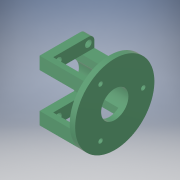
# Autodesk Inventor part: AS5047DEnclosure
Saved by Autodesk Inventor 2019.1 (Build 231200000, 200)
## iProperties
Created: 2018-06-30
Part Number: AS5047DEnclosure
Material: Generisch
Document SubType Name: Modeling
Designer: JochenAlt
Density: 1 g/cm^3
Appearance: Glatt - dunkelseegrün
Author: JochenAlt
Autodesk Inventor part; units mm, degrees
ref_plane "YZ Plane" through (0, 0, 0) normal (1, 0, 0) x (0, 1, 0)
ref_plane "XZ Plane" through (0, 0, 0) normal (0, 1, 0) x (-1, 0, 0)
ref_plane "XY Plane" through (0, 0, 0) normal (0, 0, 1) x (1, 0, 0)
ref_plane "Arbeitsebene1" through (0, 0, 0) normal (1, 0, 0) x (0, 0, -1)
sketch "Skizze1" plane through (0, 0, 0) normal (1, 0, 0) x (0, 0, -1)
  arc A0 (14.55, 0) -> (-14.55, 0) centre (0, 0) ccw
  circle A1 centre (0, 0) radius 5
  line L0 (-20.8128, 0) -> (22.3238, 0) construction
  line L1 (0, -22.3037) -> (0, 20.6923) construction
  circle A2 centre (0, 10.45) radius 0.8
  circle A3 centre (-9.05, -5.225) radius 0.8
  circle A4 centre (9.05, -5.225) radius 0.8
  circle A5 centre (0, 0) radius 10.45 construction
  line L2 (0, 0) -> (9.05, -5.225) construction
  line L3 (0, 0) -> (-9.05, -5.225) construction
  line L4 (8.89, -5.5) -> (-8.89, -5.5) construction
  line L5 (-8.89, -5.5) -> (-8.89, 5.5) construction
  line L6 (-8.89, 5.5) -> (8.89, 5.5) construction
  line L7 (8.89, 5.5) -> (8.89, -5.5) construction
  circle A6 centre (8.89, 5.5) radius 1.2
  circle A7 centre (-8.89, 5.5) radius 1.2
  arc A8 (-14.55, 0) -> (14.1469, 3.4013) centre (0, 0) ccw
  line L8 (8.89, 7.7) -> (-8.89, 7.7)
  line L9 (6.5, 3.3) -> (6.5, 7.7)
  line L10 (-4.3414, 8.5633) -> (-4.3414, 8.4781)
  line L11 (-6.5, 7.7) -> (-6.5, 3.3)
  arc A9 (3.7563, 3.3) -> (-3.7563, 3.3) centre (0, 0) ccw
  line L12 (6.5, 3.3) -> (3.7563, 3.3)
  line L13 (-3.7563, 3.3) -> (-6.5, 3.3)
  line L14 (-6.5, -9.4188) -> (-6.5, -7.4188)
  line L15 (6.5, -9.4188) -> (6.5, -7.4188)
  line L16 (11.09, -9.4188) -> (6.5, -9.4188)
  line L17 (11.09, -9.4188) -> (11.09, -7.4188)
  circle A10 centre (8.89, -5.5) radius 1.2
  circle A11 centre (-8.89, -5.5) radius 1.2
  line L18 (11.09, -7.4188) -> (11.09, 5.5)
  line L19 (-6.5, -7.4188) -> (-6.5, 3.3)
  line L20 (-11.09, -7.4188) -> (-11.09, 5.5)
  arc A12 (-8.89, 7.7) -> (-11.09, 5.5) centre (-8.89, 5.5) ccw
  arc A13 (11.09, 5.5) -> (8.89, 7.7) centre (8.89, 5.5) ccw
  arc A14 (7.715, -7.4188) -> (10.065, -7.4188) centre (8.89, -5.5) ccw
  line L21 (6.5, -7.4188) -> (7.715, -7.4188)
  line L22 (10.065, -7.4188) -> (11.09, -7.4188)
  arc A15 (-10.065, -7.4188) -> (-7.715, -7.4188) centre (-8.89, -5.5) ccw
  line L23 (-11.09, -7.4188) -> (-10.065, -7.4188)
  line L24 (-7.715, -7.4188) -> (-6.5, -7.4188)
  line L25 (6.5, -7.4188) -> (6.5, 3.3)
  line L26 (-11.09, -7.4188) -> (-11.09, -9.4188)
  line L27 (-11.09, -9.4188) -> (-6.5, -9.4188)
  point P0 (0, 14.55)
  dimension "d2" = 10
  dimension "d9" = 1.6
  dimension "d11" = 120
  dimension "d12" = 20.9
  dimension "d19" = 11
  dimension "d20" = 17.78
  dimension "d22" = 2.4
  dimension "d29" = 14.55
  dimension "d30" = 5
  dimension "d38" = 2.2
  dimension "d39" = 13
  dimension "d41" = 2
  dimension "d42" = 4.5
  constraints: 53 end point, 23 point on circle, 16 centre point, 13 coincident, 8 perpendicular, 8 point on line, 7 collinear, 7 equal radius, 6 parallel, 4 tangent, 3 horizontal, 3 vertical, 1 symmetric about line, 6 other
  measures "d2" diameter of A1
  measures "d9" diameter of A2
  measures "d11" angle of L2 L1
  measures "d12" diameter of A5
  measures "d19" distance of L4.end L5.end
  measures "d20" distance of L5.end L6.end
  measures "d22" diameter of A6
  measures "d29" radius of A8
  measures "d30" radius of A9
  measures "d38" radius of A12
  measures "d39" distance between parallel lines of L9 L11
  measures "d41" distance between parallel lines of L22 L16
  measures "d42" diameter of A14
extrude "Extrusion1" add sketch "Skizze1" against normal blind 2 contours A8 L17 L18 A13 L8 A12 L20 L26 A0 | A8 L27 L14 L19 L13 A1 L12 L25 L15 L16 | L16 L15 L21 A14 L22 L17 | L26 L23 A15 L24 L14 L27 | L22 A14 L21 L25 L9 L8 A13 L18 | L20 A12 L8 L11 L19 L24 A15 L23 | L12 A1 L13 L11 L8 L9 | A6 | A7 | A10 | A11
extrude "Extrusion3" add sketch "Skizze1" against normal blind 13.2 from surface at -2 contours L16 L15 L21 A14 L22 L17 | L26 L23 A15 L24 L14 L27 | L12 A1 L13 L11 L8 L9
extrude "Extrusion4" add sketch "Skizze1" against normal blind 3 from surface at -15.2 contours L16 L15 L21 A14 L22 L17 | L26 L23 A15 L24 L14 L27 | L22 A14 L21 L25 L9 L8 A13 L18 | L20 A12 L8 L11 L19 L24 A15 L23 | L12 A1 L13 L11 L8 L9
